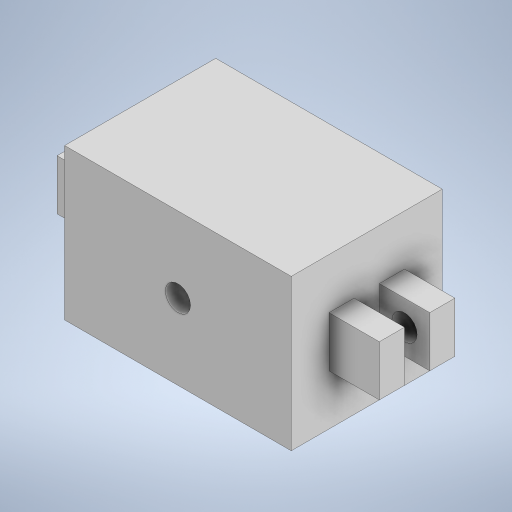
# Autodesk Inventor part: body
Saved by Autodesk Inventor 2024 (Build 280153000, 153)
## iProperties
Created: 2023-10-16
Part Number: body
Material: Generic
Document SubType Name: Modeling
Designer: Piter
Density: 1 g/cm^3
Appearance: Default
Author: Piter
Autodesk Inventor part; units mm, degrees
ref_plane "YZ Plane" through (0, 0, 0) normal (1, 0, 0) x (0, 1, 0)
ref_plane "XZ Plane" through (0, 0, 0) normal (0, 1, 0) x (-1, 0, 0)
ref_plane "XY Plane" through (0, 0, 0) normal (0, 0, 1) x (1, 0, 0)
sketch "Sketch1" plane through (0, 0, 0) normal (0, 1, 0) x (-1, 0, 0)
  line L0 (-0.2883, 0) -> (44.7117, 0)
  line L1 (44.7117, 0) -> (44.7117, 30)
  line L2 (44.7117, 30) -> (-0.2883, 30)
  line L3 (-0.2883, 30) -> (-0.2883, 0)
  point P0 (0, 0)
  dimension "d0" = 45
  dimension "d1" = 30
  constraints: 8 end point, 2 parallel, 1 horizontal, 1 perpendicular
  measures "d0" distance of L2.end L1.end
  measures "d1" distance of L1.end L0.end
extrude "Extrusion1" add sketch "Sketch1" along normal blind 30
sketch "Sketch2" plane through (-44.7117, 0, 0) normal (-1, 0, 0) x (0, 0, 1)
  line L0 (19.294, 8.1716) -> (10.706, 21.8284) construction
  line L1 (10.706, 8.1716) -> (19.294, 21.8284) construction
  line L2 (17.5, 10) -> (12.5, 10)
  line L3 (12.5, 10) -> (12.5, 20)
  line L4 (12.5, 20) -> (17.5, 20)
  line L5 (17.5, 20) -> (17.5, 10)
  line L6 (17.5, 10) -> (12.5, 20) construction
  line L7 (12.5, 10) -> (17.5, 20) construction
  line L8 (12.5, 10) -> (7.5, 10)
  line L9 (7.5, 10) -> (7.5, 20)
  line L10 (7.5, 20) -> (12.5, 20)
  line L11 (12.5, 20) -> (12.5, 10)
  line L12 (17.5, 10) -> (22.5, 10)
  line L13 (22.5, 10) -> (22.5, 20)
  line L14 (22.5, 20) -> (17.5, 20)
  line L15 (17.5, 20) -> (17.5, 10)
  point P0 (0, 0)
  point P1 (15, 15)
  dimension "d4" = 5
  dimension "d5" = 10
  dimension "d6" = 5
  dimension "d7" = 5
  constraints: 32 end point, 6 parallel, 4 midpoint, 3 horizontal, 3 perpendicular, 1 point on line
  measures "d4" distance of L3.end L4.end
  measures "d5" distance of L2.end L3.end
  measures "d6" distance of L9.end L10.end
  measures "d7" distance of L14.end L13.end
extrude "Extrusion2" add sketch "Sketch2" along normal blind 9 contours L5 L14 L13 L12 | L8 L9 L10 L3
sketch "Sketch3" plane through (-44.7117, 10, 7.5) normal (0, 0, -1) x (-1, 0, 0)
  line L0 (0, -10) -> (0, 20) projected
  line L1 (0, 5) -> (5, 5)
  circle A0 centre (5, 5) radius 2.5
  point P0 (-44.7117, -10)
  dimension "d10" = 5
  dimension "d11" = 5
  constraints: 2 end point, 1 centre point, 1 coincident, 1 horizontal, 1 midpoint
  measures "d10" distance of L1.start L1.end
  measures "d11" diameter of A0
extrude "Extrusion3" cut sketch "Sketch3" against normal through all
sketch "Sketch4" plane through (0.2883, 0, 30) normal (1, 0, 0) x (0, 0, -1)
  line L0 (12.5, 10) -> (12.5, 20) projected
  line L1 (17.5, 10) -> (22.5, 10) projected
  line L2 (12.5, 20) -> (17.5, 20)
  line L3 (17.5, 20) -> (17.5, 10)
  line L4 (17.5, 10) -> (12.5, 10)
  line L5 (12.5, 10) -> (12.5, 20)
  line L6 (17.5, 20) -> (22.5, 20) projected
  line L7 (17.5, 10) -> (22.5, 10)
  line L8 (22.5, 10) -> (22.5, 20)
  line L9 (22.5, 20) -> (17.5, 20)
  line L10 (17.5, 20) -> (17.5, 10)
  line L11 (7.5, 10) -> (12.5, 10) projected
  line L12 (12.5, 20) -> (7.5, 20)
  line L13 (7.5, 20) -> (7.5, 10)
  line L14 (7.5, 10) -> (12.5, 10)
  line L15 (12.5, 10) -> (12.5, 20)
  point P0 (30, 0)
  constraints: 24 end point, 6 parallel, 3 horizontal, 3 perpendicular
extrude "Extrusion4" add sketch "Sketch4" along normal blind 10 contours L11 L13 L12 L0 | L3 L6 L8 L1
sketch "Sketch5" plane through (0.2883, 10, 12.5) normal (0, 0, 1) x (-1, 0, 0)
  line L0 (0, 10) -> (0, -20) projected
  line L1 (0, -5) -> (-5, -5)
  circle A0 centre (-5, -5) radius 2.5
  point P0 (0.2883, 10)
  dimension "d16" = 5
  dimension "d17" = 5
  constraints: 2 end point, 1 centre point, 1 coincident, 1 horizontal, 1 midpoint
  measures "d16" distance of L1.start L1.end
  measures "d17" diameter of A0
extrude "Extrusion5" cut sketch "Sketch5" against normal through all
sketch "Sketch6" plane through (-44.7117, 0, 30) normal (0, 0, 1) x (1, 0, 0)
  circle A0 centre (22.5, 15) radius 2.5
  line L0 (0, 0) -> (0, 30) projected
  point P0 (44.7117, 0)
  point P1 (0, 15)
  dimension "d20" = 5
  dimension "d23" = 22.5
  constraints: 1 centre point, 1 midpoint
  measures "d20" diameter of A0
  measures "d23" distance of point (0, 15) A0.centre
extrude "Extrusion6" cut sketch "Sketch6" against normal blind 5
body "Solid1"
